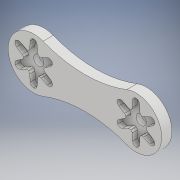
# Autodesk Inventor part: Pata - Antebrazo
Saved by Autodesk Inventor 2019 (Build 230136000, 136)
## iProperties
Created: 2020-02-11
Part Number: Pata - Antebrazo
Material: ABS Plastic
Document SubType Name: Modeling
Designer: jacqu
Density: 1.06 g/cm^3
Appearance: Smooth - White
Mass: 6.28509 g
Surface Area: 55.6042 cm^2
Volume: 5.92933 cm^3
d0: 20.000 mm
Author: jacqu
Autodesk Inventor part; units mm, degrees
ref_plane "YZ Plane" through (0, 0, 0) normal (1, 0, 0) x (0, 1, 0)
ref_plane "XZ Plane" through (0, 0, 0) normal (0, 1, 0) x (-1, 0, 0)
ref_plane "XY Plane" through (0, 0, 0) normal (0, 0, 1) x (1, 0, 0)
sketch "Sketch1" plane through (0, 0, 0) normal (0, 0, 1) x (1, 0, 0)
  arc A0 (-72.7273, 18.6308) -> (-72.7273, -18.6308) centre (-80, 0) ccw
  arc A1 (-7.2727, -18.6308) -> (-72.7273, -18.6308) centre (-40, -102.4695) ccw
  arc A2 (-7.2727, -18.6308) -> (-7.2727, 18.6308) centre (0, 0) ccw
  arc A3 (-72.7273, 18.6308) -> (-7.2727, 18.6308) centre (-40, 102.4695) ccw
  arc A4 (-79.5765, 3.9775) -> (-79.5765, -3.9775) centre (-80, 0) ccw
  arc A5 (-0.4235, -3.9775) -> (-0.4235, 3.9775) centre (0, 0) ccw
  arc A6 (-80.4235, -3.9775) -> (-80.4235, 3.9775) centre (-80, 0) ccw
  arc A7 (-0.4235, 3.9775) -> (-0.4235, -3.9775) centre (0, 0) ccw
  point P0 (-103.8261, -115.9088)
  dimension "d0" = 20
  dimension "d1" = 20
  dimension "d2" = 90
  dimension "d3" = 90
  dimension "d4" = 4
  dimension "d7" = 80
  dimension "d33" = 4
  constraints: 18 point on circle, 8 centre point, 6 tangent, 3 coincident, 2 equal radius, 1 horizontal alignment
  measures "d0" radius of A0
  measures "d1" radius of A2
  measures "d2" radius of A3
  measures "d3" radius of A1
  measures "d4" radius of A4
  measures "d7" distance of A5.centre A4.centre
  measures "d33" radius of A6
extrude "Extrusion1" add sketch "Sketch1" along normal blind 8 contours A3 A2 A1 A0 | A6 A4 | A7 A5
sketch "Sketch3" plane through (0, 0, 8) normal (0, 0, 1) x (1, 0, 0)
  arc A0 (-72.7273, 18.6308) -> (-72.7273, -18.6308) centre (-80, 0) ccw projected
  arc A1 (-7.2727, -18.6308) -> (-72.7273, -18.6308) centre (-40, -102.4695) ccw projected
  arc A2 (-7.2727, -18.6308) -> (-7.2727, 18.6308) centre (0, 0) ccw projected
  arc A3 (-72.7273, 18.6308) -> (-7.2727, 18.6308) centre (-40, 102.4695) ccw projected
  line L0 (-56.02, 2) -> (-23.98, 2)
  line L1 (-56.02, -2) -> (-23.98, -2)
  arc A4 (-56.02, 2) -> (-56.02, -2) centre (-56.02, 0) ccw
  arc A5 (-23.98, -2) -> (-23.98, 2) centre (-23.98, 0) ccw
  point P0 (-83.48, 0)
  dimension "d12" = 2
  constraints: 4 end point, 4 point on circle, 4 tangent, 2 centre point, 2 horizontal, 1 horizontal alignment
  measures "d12" radius of A4
extrude "Extrusion2" cut sketch "Sketch3" against normal blind 6 contours L0 A5 L1 A4
ref_plane "Work Plane2" through (-40, 0, 8) normal (-1, 0, 0) x (0, -1, 0)
ref_plane "Work Plane1" through (-100, 0, 8) normal (-1, 0, 0) x (0, -1, 0)
sketch "Sketch8" plane through (0, 0, 0) normal (0, 0, -1) x (-1, 0, 0)
  arc A0 (-5.9847, 6.9335) -> (-4.1961, 6.8112) centre (-4.9584, 8.8037) ccw
  arc A1 (-5.9847, 6.9335) -> (-10.6867, 9.2491) centre (-34.4674, -44.9687) ccw
  arc A2 (-10.6867, 9.2491) -> (-14.3183, 8.2667) centre (-11.9528, 6.7261) ccw
  arc A3 (-14.3183, 8.2667) -> (-13.3533, 4.6303) centre (-11.8014, 6.9884) ccw
  arc A4 (-13.3533, 4.6303) -> (-8.9969, 1.7162) centre (21.7104, 52.334) ccw
  arc A5 (-7.9967, 0.2284) -> (-8.9969, 1.7162) centre (-10.1034, -0.1078) ccw
  arc A6 (-7.9967, 0.2284) -> (-7.9967, -0.2284) centre (0, 0) ccw
  arc A7 (-8.9969, -1.7162) -> (-7.9967, -0.2284) centre (-10.1034, 0.1078) ccw
  arc A8 (-8.9969, -1.7162) -> (-13.3533, -4.6303) centre (21.7104, -52.334) ccw
  arc A9 (-13.3533, -4.6303) -> (-14.3183, -8.2667) centre (-11.8014, -6.9884) ccw
  arc A10 (-14.3183, -8.2667) -> (-10.6867, -9.2491) centre (-11.9528, -6.7261) ccw
  arc A11 (-10.6867, -9.2491) -> (-5.9847, -6.9335) centre (-34.4674, 44.9687) ccw
  arc A12 (-4.1961, -6.8112) -> (-5.9847, -6.9335) centre (-4.9584, -8.8037) ccw
  arc A13 (-4.1961, -6.8112) -> (-3.8006, -7.0396) centre (0, 0) ccw
  arc A14 (-3.0122, -8.6497) -> (-3.8006, -7.0396) centre (-5.145, -8.6959) ccw
  arc A15 (-3.0122, -8.6497) -> (-2.6667, -13.8795) centre (56.1778, -7.3653) ccw
  arc A16 (-2.6667, -13.8795) -> (0, -16.5333) centre (0.1514, -13.7145) ccw
  arc A17 (0, -16.5333) -> (2.6667, -13.8795) centre (-0.1514, -13.7145) ccw
  arc A18 (2.6667, -13.8795) -> (3.0122, -8.6497) centre (-56.1778, -7.3653) ccw
  arc A19 (3.8006, -7.0396) -> (3.0122, -8.6497) centre (5.145, -8.6959) ccw
  arc A20 (3.8006, -7.0396) -> (4.1961, -6.8112) centre (0, 0) ccw
  arc A21 (5.9847, -6.9335) -> (4.1961, -6.8112) centre (4.9584, -8.8037) ccw
  arc A22 (5.9847, -6.9335) -> (10.6867, -9.2491) centre (34.4674, 44.9687) ccw
  arc A23 (10.6867, -9.2491) -> (14.3183, -8.2667) centre (11.9528, -6.7261) ccw
  arc A24 (14.3183, -8.2667) -> (13.3533, -4.6303) centre (11.8014, -6.9884) ccw
  arc A25 (13.3533, -4.6303) -> (8.9969, -1.7162) centre (-21.7104, -52.334) ccw
  arc A26 (7.9967, -0.2284) -> (8.9969, -1.7162) centre (10.1034, 0.1078) ccw
  arc A27 (7.9967, -0.2284) -> (7.9967, 0.2284) centre (0, 0) ccw
  arc A28 (8.9969, 1.7162) -> (7.9967, 0.2284) centre (10.1034, -0.1078) ccw
  arc A29 (8.9969, 1.7162) -> (13.3533, 4.6303) centre (-21.7104, 52.334) ccw
  arc A30 (13.3533, 4.6303) -> (14.3183, 8.2667) centre (11.8014, 6.9884) ccw
  arc A31 (14.3183, 8.2667) -> (10.6867, 9.2491) centre (11.9528, 6.7261) ccw
  arc A32 (10.6867, 9.2491) -> (5.9847, 6.9335) centre (34.4674, -44.9687) ccw
  arc A33 (4.1961, 6.8112) -> (5.9847, 6.9335) centre (4.9584, 8.8037) ccw
  arc A34 (4.1961, 6.8112) -> (3.8006, 7.0396) centre (0, 0) ccw
  arc A35 (3.0122, 8.6497) -> (3.8006, 7.0396) centre (5.145, 8.6959) ccw
  arc A36 (3.0122, 8.6497) -> (2.6667, 13.8795) centre (-56.1778, 7.3653) ccw
  arc A37 (2.6667, 13.8795) -> (0, 16.5333) centre (-0.1514, 13.7145) ccw
  arc A38 (0, 16.5333) -> (-2.6667, 13.8795) centre (0.1514, 13.7145) ccw
  arc A39 (-2.6667, 13.8795) -> (-3.0122, 8.6497) centre (56.1778, 7.3653) ccw
  arc A40 (-3.8006, 7.0396) -> (-3.0122, 8.6497) centre (-5.145, 8.6959) ccw
  arc A41 (-3.8006, 7.0396) -> (-4.1961, 6.8112) centre (0, 0) ccw
  circle A42 centre (0, 0) radius 4
  arc A43 (10.6867, -9.2491) -> (14.3183, -8.2667) centre (11.9528, -6.7261) ccw
  arc A44 (0, -16.5333) -> (2.6667, -13.8795) centre (-0.1514, -13.7145) ccw
  dimension "d39" = 8
  constraints: 88 point on circle, 45 centre point
  measures "d39" diameter of A42
sketch "Sketch9" plane through (0, 0, 0) normal (0, 0, -1) x (-1, 0, 0)
  circle A0 centre (-6.9282, -4) radius 0.5333
  circle A1 centre (-6.9282, 4) radius 0.5333
  circle A2 centre (6.9282, 4) radius 0.5333
  circle A3 centre (6.9282, -4) radius 0.5333
  arc A4 (-5.9847, 6.9335) -> (-4.1961, 6.8112) centre (-4.9584, 8.8037) ccw
  arc A5 (-5.9847, 6.9335) -> (-10.6867, 9.2491) centre (-34.4674, -44.9687) ccw
  arc A6 (-10.6867, 9.2491) -> (-14.3183, 8.2667) centre (-11.9528, 6.7261) ccw
  arc A7 (-14.3183, 8.2667) -> (-13.3533, 4.6303) centre (-11.8014, 6.9884) ccw
  arc A8 (-13.3533, 4.6303) -> (-8.9969, 1.7162) centre (21.7104, 52.334) ccw
  arc A9 (-7.9967, 0.2284) -> (-8.9969, 1.7162) centre (-10.1034, -0.1078) ccw
  arc A10 (-7.9967, 0.2284) -> (-7.9967, -0.2284) centre (0, 0) ccw
  arc A11 (-8.9969, -1.7162) -> (-7.9967, -0.2284) centre (-10.1034, 0.1078) ccw
  arc A12 (-8.9969, -1.7162) -> (-13.3533, -4.6303) centre (21.7104, -52.334) ccw
  arc A13 (-13.3533, -4.6303) -> (-14.3183, -8.2667) centre (-11.8014, -6.9884) ccw
  arc A14 (-14.3183, -8.2667) -> (-10.6867, -9.2491) centre (-11.9528, -6.7261) ccw
  arc A15 (-10.6867, -9.2491) -> (-5.9847, -6.9335) centre (-34.4674, 44.9687) ccw
  arc A16 (-4.1961, -6.8112) -> (-5.9847, -6.9335) centre (-4.9584, -8.8037) ccw
  arc A17 (-4.1961, -6.8112) -> (-3.8006, -7.0396) centre (0, 0) ccw
  arc A18 (-3.0122, -8.6497) -> (-3.8006, -7.0396) centre (-5.145, -8.6959) ccw
  arc A19 (-3.0122, -8.6497) -> (-2.6667, -13.8795) centre (56.1778, -7.3653) ccw
  arc A20 (-2.6667, -13.8795) -> (0, -16.5333) centre (0.1514, -13.7145) ccw
  arc A21 (0, -16.5333) -> (2.6667, -13.8795) centre (-0.1514, -13.7145) ccw
  arc A22 (2.6667, -13.8795) -> (3.0122, -8.6497) centre (-56.1778, -7.3653) ccw
  arc A23 (3.8006, -7.0396) -> (3.0122, -8.6497) centre (5.145, -8.6959) ccw
  arc A24 (3.8006, -7.0396) -> (4.1961, -6.8112) centre (0, 0) ccw
  arc A25 (5.9847, -6.9335) -> (4.1961, -6.8112) centre (4.9584, -8.8037) ccw
  arc A26 (5.9847, -6.9335) -> (10.6867, -9.2491) centre (34.4674, 44.9687) ccw
  arc A27 (10.6867, -9.2491) -> (14.3183, -8.2667) centre (11.9528, -6.7261) ccw
  arc A28 (14.3183, -8.2667) -> (13.3533, -4.6303) centre (11.8014, -6.9884) ccw
  arc A29 (13.3533, -4.6303) -> (8.9969, -1.7162) centre (-21.7104, -52.334) ccw
  arc A30 (7.9967, -0.2284) -> (8.9969, -1.7162) centre (10.1034, 0.1078) ccw
  arc A31 (7.9967, -0.2284) -> (7.9967, 0.2284) centre (0, 0) ccw
  arc A32 (8.9969, 1.7162) -> (7.9967, 0.2284) centre (10.1034, -0.1078) ccw
  arc A33 (8.9969, 1.7162) -> (13.3533, 4.6303) centre (-21.7104, 52.334) ccw
  arc A34 (13.3533, 4.6303) -> (14.3183, 8.2667) centre (11.8014, 6.9884) ccw
  arc A35 (14.3183, 8.2667) -> (10.6867, 9.2491) centre (11.9528, 6.7261) ccw
  arc A36 (10.6867, 9.2491) -> (5.9847, 6.9335) centre (34.4674, -44.9687) ccw
  arc A37 (4.1961, 6.8112) -> (5.9847, 6.9335) centre (4.9584, 8.8037) ccw
  arc A38 (4.1961, 6.8112) -> (3.8006, 7.0396) centre (0, 0) ccw
  arc A39 (3.0122, 8.6497) -> (3.8006, 7.0396) centre (5.145, 8.6959) ccw
  arc A40 (3.0122, 8.6497) -> (2.6667, 13.8795) centre (-56.1778, 7.3653) ccw
  arc A41 (2.6667, 13.8795) -> (0, 16.5333) centre (-0.1514, 13.7145) ccw
  arc A42 (0, 16.5333) -> (-2.6667, 13.8795) centre (0.1514, 13.7145) ccw
  arc A43 (-2.6667, 13.8795) -> (-3.0122, 8.6497) centre (56.1778, 7.3653) ccw
  arc A44 (-3.8006, 7.0396) -> (-3.0122, 8.6497) centre (-5.145, 8.6959) ccw
  arc A45 (-3.8006, 7.0396) -> (-4.1961, 6.8112) centre (0, 0) ccw
  circle A46 centre (0, 0) radius 4
  arc A47 (10.6867, -9.2491) -> (14.3183, -8.2667) centre (11.9528, -6.7261) ccw
  arc A48 (0, -16.5333) -> (2.6667, -13.8795) centre (-0.1514, -13.7145) ccw
  dimension "d40" = 8
  constraints: 88 point on circle, 49 centre point
  measures "d40" diameter of A46
extrude "Extrusion6" cut sketch "Sketch8" against normal blind 4
sketch "Sketch10" plane through (0, 0, 0) normal (0, 0, -1) x (-1, 0, 0)
  circle A0 centre (0, 0) radius 4
  dimension "d43" = 8
  constraints: 1 centre point, 1 coincident
  measures "d43" diameter of A0
extrude "Extrusion7" cut sketch "Sketch10" against normal blind 10
mirror "Mirror4" about plane through (-40, 0, 8) normal (-1, 0, 0) of "Extrusion6", "Extrusion7"
equation "\"d0\" = radio_muslo"
equation "\"d1\" = d0"
equation "\"d2\" = curva"
equation "\"d3\" = d2"
equation "\"d4\" = 0.5 * diametro_servo"
equation "\"d7\" = distancia_centros"
equation "\"d33\" = d4"
equation "\"d39\" = diametro_servo"
equation "\"d43\" = diametro_servo"
equation "\"curva\" = 90"
equation "\"distancia_centros\" = 80"
equation "\"espesor\" = 3.3"
equation "\"diametro_servo\" = 8"
equation "\"radio_muslo\" = 20"
body "Solid1"
